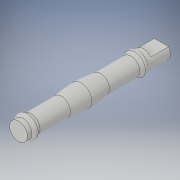
# Autodesk Inventor part: Рукаядь рукоядки
Saved by Autodesk Inventor 2019 (Build 230136000, 136)
## iProperties
Created: 2019-04-28
Part Number: Рукаядь рукоядки
Material: Типовые
Document SubType Name: Modeling
Designer: BarmanKaktus
Density: 1 g/cm^3
Appearance: По умолчанию
Author: BarmanKaktus
Autodesk Inventor part; units mm, degrees
ref_plane "YZ Plane" through (0, 0, 0) normal (1, 0, 0) x (0, 1, 0)
ref_plane "XY Plane" through (0, 0, 0) normal (0, 0, 1) x (1, 0, 0)
sketch "Эскиз1" plane through (0, 0, 0) normal (0, 0, 1) x (1, 0, 0)
  circle A0 centre (0, 0) radius 5
  dimension "d0" = 10
  constraints: 1 centre point, 1 coincident
  measures "d0" diameter of A0
extrude "Выдавливание1" add sketch "Эскиз1" along normal blind 80
sketch "Эскиз2" plane through (0, 0, 0) normal (0, 0, -1) x (-1, 0, 0)
  line L0 (0, 0) -> (0, 3)
  line L1 (0, 3) -> (-4, 3)
  circle A0 centre (0, 0) radius 5 projected
  line L2 (4, 3) -> (0, 3)
  constraints: 6 end point, 2 point on circle, 1 collinear, 1 point on line, 1 vertical
extrude "Выдавливание2" cut sketch "Эскиз2" against normal blind 10 contours L1 A0 L2 picked at (-2.4012, 3.2796)
ref_plane "РабПлоскость1" through (0, 0, 0) normal (0, 1, 0) x (-1, 0, 0)
sketch "Эскиз3" plane through (0, 0, 0) normal (0, 1, 0) x (-1, 0, 0)
  line L0 (0, 10) -> (0, 80)
  line L1 (5, 80) -> (-5, 80) projected
  line L2 (0, 10) -> (0, 15)
  line L3 (0, 15) -> (6, 15)
  line L4 (0, 15) -> (0, 20)
  line L5 (0, 20) -> (4, 20)
  line L6 (0, 20) -> (0, 45)
  line L7 (0, 45) -> (0, 70)
  line L8 (0, 70) -> (4, 70)
  line L9 (0, 70) -> (0, 75)
  line L10 (0, 75) -> (6, 75)
  line L11 (0, 45) -> (6, 45)
  spline S0 degree 4 poles (0, 80) (13.7387, 74.1571) (-5.0029, 77.0727) (17.394, 45) (-5.0029, 12.9273) (13.7387, 15.8429) (0, 10) knots 0 0 0 0 0 0.409508 0.590492 1 1 1 1 1
  point P0 (0, 0)
  dimension "d7" = 5
  dimension "d8" = 6
  dimension "d9" = 5
  dimension "d10" = 4
  dimension "d11" = 25
  dimension "d12" = 25
  dimension "d13" = 4
  constraints: 22 end point, 4 point on line, 3 perpendicular, 2 horizontal, 2 midpoint, 7 other
  measures "d7" distance of L0.start L2.end
  measures "d8" distance of L2.end L3.end
  measures "d9" distance of L2.end L4.end
  measures "d10" distance of L4.end L5.end
  measures "d11" distance of L4.end L6.end
  measures "d12" distance of L6.end L7.end
  measures "d13" distance of L7.end L8.end
revolve "Вращение1" add sketch "Эскиз3" angle 360 about axis through (0, 0, 10) along (0, 0, 1)
